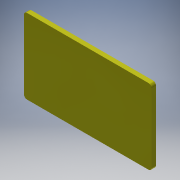
# Autodesk Inventor part: kaart
Saved by Autodesk Inventor 2019 (Build 230136000, 136)
## iProperties
Created: 2020-06-08
Part Number: kaart
Material: Generic
Document SubType Name: Modeling
Designer: Jaap Kort
Density: 1 g/cm^3
Appearance: Yellow
Author: Jaap Kort
Autodesk Inventor part; units mm, degrees
ref_plane "YZ Plane" through (0, 0, 0) normal (1, 0, 0) x (0, 1, 0)
ref_plane "XZ Plane" through (0, 0, 0) normal (0, 1, 0) x (-1, 0, 0)
ref_plane "XY Plane" through (0, 0, 0) normal (0, 0, 1) x (1, 0, 0)
sketch "Sketch1" plane through (0, 0, 0) normal (0, 0, 1) x (1, 0, 0)
  line L0 (42.5, 25) -> (-42.5, 25)
  line L1 (-42.5, 25) -> (-42.5, -25)
  line L2 (-42.5, -25) -> (42.5, -25)
  line L3 (42.5, -25) -> (42.5, 25)
  line L4 (42.5, 25) -> (-42.5, -25) construction
  line L5 (-42.5, 25) -> (42.5, -25) construction
  point P0 (0, 0)
  dimension "d5" = 85
  dimension "d6" = 50
  constraints: 12 end point, 2 midpoint, 2 parallel, 1 horizontal, 1 perpendicular
  measures "d5" distance of L2.end L1.end
  measures "d6" distance of L1.end L0.end
extrude "Extrusion1" add sketch "Sketch1" along normal blind 3
fillet "Fillet1" radius 2 4 edges at (-42.5, 25, 1.5) (-42.5, -25, 1.5) (42.5, 25, 1.5) (42.5, -25, 1.5)
body "Solid1"
